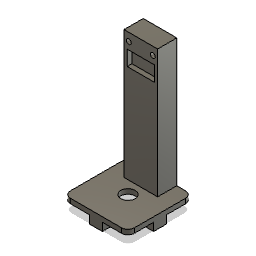
splicer_sample-fixation_003 (Autodesk Fusion 360 design; units mm, degrees)
Autodesk Fusion 360 part; units mm, degrees
sketch "Sketch1" plane through (0, 0, 0) normal (0, 1, 0) x (1, 0, 0)
  line L0 (20, -20) -> (-20, -20)
  line L1 (-20, -20) -> (-20, 20)
  line L2 (-20, 20) -> (20, 20)
  line L3 (20, 20) -> (20, -20)
  line L4 (20, -20) -> (-20, 20) construction
  line L5 (-20, -20) -> (20, 20) construction
  line L6 (-20, 4) -> (-15, 4)
  line L7 (-15, 4) -> (-15, -4)
  line L8 (-15, -4) -> (-20, -4)
  line L9 (-20, -4) -> (-20, 4)
  line L10 (-4, 20) -> (4, 20)
  line L11 (4, 20) -> (4, 15)
  line L12 (4, 15) -> (-4, 15)
  line L13 (-4, 15) -> (-4, 20)
  line L14 (20, 4) -> (15, 4)
  line L15 (15, 4) -> (15, -4)
  line L16 (15, -4) -> (20, -4)
  line L17 (20, -4) -> (20, 4)
  line L18 (-4, -20) -> (4, -20)
  line L19 (4, -20) -> (4, -15)
  line L20 (4, -15) -> (-4, -15)
  line L21 (-4, -15) -> (-4, -20)
  dimension "d1" = 40
  dimension "d2" = 40
  dimension "d3" = 5
  dimension "d4" = 8
  dimension "d5" = 16
  dimension "d6" = 5
  dimension "d7" = 16
  dimension "d8" = 8
  dimension "d9" = 5
  dimension "d10" = 5
  dimension "d11" = 8
  dimension "d12" = 8
  dimension "d13" = 16
  dimension "d14" = 16
  constraint horizontal L0
  constraint perpendicular L0 L1
  constraint parallel L0 L2
  constraint parallel L1 L3
  constraint coincident L4 origin
  constraint coincident L5 origin
  constraint horizontal L6
  constraint vertical L7
  constraint horizontal L8
  constraint vertical L9
  constraint coincident L1 L6.start
  constraint horizontal L10
  constraint vertical L11
  constraint horizontal L12
  constraint vertical L13
  constraint coincident L2 L10.start
  constraint horizontal L14
  constraint vertical L15
  constraint horizontal L16
  constraint vertical L17
  constraint coincident L3 L14.start
  constraint horizontal L18
  constraint vertical L19
  constraint horizontal L20
  constraint vertical L21
  constraint coincident L0 L18.start
  measures "d1" distance of L1.end L2.end
  measures "d2" distance of L0.end L1.end
  measures "d3" distance of L6.start L6.end
  measures "d4" distance of L6.start L8.end
  measures "d5" distance of L1.end L6.start
  measures "d6" distance of L10.start L12.end
  measures "d7" distance of L1.end L10.start
  measures "d8" distance of L11 L13
  measures "d9" distance of L18.start L20.end
  measures "d10" distance of L14.start L14.end
  measures "d11" distance of L14.end L15.end
  measures "d12" distance of L19.end L20.end
  measures "d13" distance of L1 L21
  measures "d14" distance of L0.start L16
extrude "Extrude1" add sketch "Sketch1" against normal blind 3 contours L0 L1 L2 L3 L6 L7 L8 L11 L12 L13 L14 L15 L16 L19 L20 L21
extrude "Extrude2" add sketch "Sketch1" against normal blind 8 contours L0 L18 L19 L20 L21 | L3 L14 L15 L16 L17 | L1 L6 L7 L8 L9 | L2 L10 L11 L12 L13
hole "Hole1" at (0, 0, 0) direction (0, -1, 0) diameter 9 depth 30 tip angle 118
fillet "Fillet1" radius 4 4 edges at (20, -1.5, -20) (-20, -1.5, -20) (20, -1.5, 20) (-20, -1.5, 20)
sketch "Sketch2" plane through (0, 0, 0) normal (0, 0, 1) x (1, 0, 0)
sketch "Sketch3" plane through (0, 0, 0) normal (0, 1, 0) x (1, 0, 0)
  line L0 (-10.5, 20) -> (10.5, 20)
  line L1 (10.5, 20) -> (10.5, 8)
  line L2 (10.5, 8) -> (-10.5, 8)
  line L3 (-10.5, 8) -> (-10.5, 20)
  line L4 (-20, -20) -> (-20, 20)
  dimension "d26" = 21
  dimension "d27" = 9.5
  dimension "d28" = 12
  constraint horizontal L0
  constraint vertical L1
  constraint horizontal L2
  constraint vertical L3
  measures "d26" distance of L1.end L2.end
  measures "d27" distance of L3 L4
  measures "d28" distance of L0.end L1.end
extrude "Extrude3" add sketch "Sketch3" along normal blind 80
sketch "Sketch4" plane through (0, 0, -8) normal (0, 0, 1) x (1, 0, 0)
  line L0 (-10.5, 0) -> (10.5, 0)
  line L1 (10.5, 0) -> (10.5, 80)
  line L2 (10.5, 80) -> (-10.5, 80)
  line L3 (-10.5, 80) -> (-10.5, 0)
  line L4 (-10.5, 80) -> (10.5, 80)
  line L5 (10.5, 80) -> (10.5, 59)
  line L6 (10.5, 59) -> (-10.5, 59)
  line L7 (-10.5, 59) -> (-10.5, 80)
  line L8 (8.5, 78) -> (8.5, 61)
  line L9 (8.5, 61) -> (-8.5, 61)
  line L10 (-8.5, 61) -> (-8.5, 78)
  line L11 (-8.5, 78) -> (8.5, 78)
  line L12 (-8.5, 78) -> (8.5, 78)
  line L13 (8.5, 78) -> (8.5, 64.8708)
  line L14 (-8.5, 64.8708) -> (-8.5, 78)
  line L15 (-8.5, 61) -> (8.5, 61)
  line L16 (8.5, 61) -> (8.5, 70.3993)
  line L17 (8.5, 70.3993) -> (-8.5, 70.3993)
  line L18 (-8.5, 70.3993) -> (-8.5, 61)
  point P0 (-7.5, 64)
  point P1 (7.5, 64)
  dimension "d29" = 21
  dimension "d30" = 21
  dimension "d31" = 2
  dimension "d34" = 5
  dimension "d35" = 15
  dimension "d36" = 3
  constraint horizontal L4
  constraint vertical L5
  constraint horizontal L6
  constraint vertical L7
  constraint coincident L2.end L3.start
  constraint horizontal L12
  constraint vertical L13
  constraint vertical L14
  constraint coincident L8 L13.end
  constraint horizontal P0 P1
  constraint horizontal L15
  constraint vertical L16
  constraint horizontal L17
  constraint vertical L18
  constraint coincident L13 L16.end
  measures "d29" distance of L2.end L1.end
  measures "d30" distance of L2.end L6.end
  measures "d34" distance of L6 P0
  measures "d35" distance of P0 P1
  measures "d36" distance of L7 P0
extrude "Extrude5" cut sketch "Sketch4" against normal blind 3 contours L8 L9 L10 L13 L14 L15 L16 L17 L18
sketch "Sketch6" plane through (0, 0, -20) normal (0, 0, -1) x (-1, 0, 0)
  line L0 (16, -3) -> (16, 0)
  line L1 (16, 0) -> (10.5, 0)
  line L2 (10.5, 0) -> (10.5, 80)
  line L3 (10.5, 80) -> (-10.5, 80)
  line L4 (-10.5, 80) -> (-10.5, 0)
  line L5 (-10.5, 0) -> (-16, 0)
  line L6 (-16, 0) -> (-16, -3)
  line L7 (-16, -3) -> (-4, -3)
  line L8 (-4, -3) -> (-4, -8)
  line L9 (-4, -8) -> (4, -8)
  line L10 (4, -8) -> (4, -3)
  line L11 (4, -3) -> (16, -3)
  point P0 (-7.5, 75)
  point P1 (7.5, 75)
  dimension "d45" = 15
  dimension "d46" = 3
  dimension "d47" = 5
  constraint horizontal P0 P1
  measures "d45" distance of P0 P1
  measures "d46" distance of L4 P0
  measures "d47" distance of L3 P0
hole "Hole4" at (7.5, 75, -20) at (-7.5, 75, -20) direction (0, 0, 1) diameter 3 depth 12 tip angle 118 counterbore diameter 5 counterbore depth 9
equation "d6 = d3"
equation "d7 = d5"
equation "d8 = d4"
equation "d9 = d3"
equation "d10 = d3"
equation "d11 = d4"
equation "d12 = d4"
equation "d13 = d7"
equation "d14 = d7"
named bodies: "4040_fixation_base"
